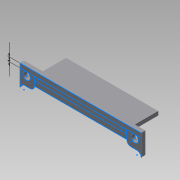
# Autodesk Inventor part: pelindung uvtron
Saved by Autodesk Inventor 2015 SP1 (Build 190203100, 203)
## iProperties
Created: 2015-04-21
Part Number: pelindung uvtron
Material: Generic
Document SubType Name: Modeling
Designer: Rafi Kurnia Putra
Density: 1 g/cm^3
Appearance: Default
Author: Rafi Kurnia Putra
Autodesk Inventor part; units mm, degrees
ref_plane "YZ Plane" through (0, 0, 0) normal (1, 0, 0) x (0, 1, 0)
ref_plane "XZ Plane" through (0, 0, 0) normal (0, 1, 0) x (-1, 0, 0)
ref_plane "XY Plane" through (0, 0, 0) normal (0, 0, 1) x (1, 0, 0)
sketch "Sketch1" plane through (0, 0, 0) normal (0, 1, 0) x (-1, 0, 0)
  circle A0 centre (25.5, 34.24) radius 1.75
  circle A1 centre (-25.5, 34.24) radius 1.75
  line L0 (23.7877, 30) -> (26.625, 30)
  arc A2 (21.7877, 32) -> (23.7877, 30) centre (23.7877, 32) ccw
  line L1 (21.7877, 35.55) -> (21.7877, 32)
  arc A3 (21.7877, 35.55) -> (21.7387, 35.99) centre (19.7877, 35.55) ccw
  arc A4 (28.625, 28) -> (26.625, 30) centre (26.625, 28) ccw
  line L2 (-21.7877, 32) -> (-21.7877, 35.55)
  arc A5 (-21.7387, 35.99) -> (-21.7877, 35.55) centre (-19.7877, 35.55) ccw
  arc A6 (-23.7877, 30) -> (-21.7877, 32) centre (-23.7877, 32) ccw
  line L3 (-26.625, 30) -> (-23.7877, 30)
  arc A7 (-26.625, 30) -> (-28.625, 28) centre (-26.625, 28) ccw
  line L4 (28.625, 28) -> (28.625, 35.99)
  line L5 (-28.625, 28) -> (-28.625, 35.99)
  line L6 (21.7877, 34.24) -> (-21.7877, 34.24)
  line L7 (28.625, 35.99) -> (-28.625, 35.99)
  line L8 (21.7877, 32) -> (-21.7877, 32)
  line L9 (-28.625, 35.99) -> (28.625, 35.99)
  line L10 (28.625, 35.99) -> (28.625, 37.99)
  line L11 (28.625, 37.99) -> (-28.625, 37.99)
  line L12 (-28.625, 37.99) -> (-28.625, 35.99)
  dimension "d6" = 2
  constraints: 26 end point, 12 point on circle, 8 centre point, 4 point on line, 3 parallel, 2 horizontal, 2 perpendicular, 2 vertical, 1 tangent
  measures "d6" distance of L10.end L9.end
extrude "Extrusion1" add sketch "Sketch1" along normal blind 2 contours L7 L4 A4 L0 A2 L1 A3 | A5 L2 A6 L3 A7 L5 L7
extrude "Extrusion2" add sketch "Sketch1" along normal blind 15 contours A3 L1 L6 L2 A5 L7
extrude "Extrusion3" add sketch "Sketch1" along normal blind 1 contours L1 L8 L2 L6
extrude "Extrusion4" add sketch "Sketch1" along normal blind 2 contours L7 L12 L11 L10
body "Solid1"
